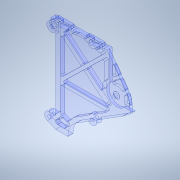
# Autodesk Inventor part: 後ろウィング固定フレームver2(ミラー)
Saved by Autodesk Inventor 2020.2 (Build 242310000, 310)
## iProperties
Created: 2020-05-07
Part Number: 後ろウィング固定フレームver2(ミラー)
Material: ポリカーボネート、クリア
Document SubType Name: Modeling
Designer: mozar
Density: 1.2 g/cm^3
Appearance: ポリカーボネート - クリア
Mass: 16.2166 g
Surface Area: 139.125 cm^2
Volume: 13.5139 cm^3
Author: mozar
Autodesk Inventor part; units mm, degrees
(part 1 of 4)
ref_plane "YZ Plane" through (0, 0, 0) normal (1, 0, 0) x (0, 1, 0)
ref_plane "XZ Plane" through (0, 0, 0) normal (0, 1, 0) x (-1, 0, 0)
ref_plane "XY Plane" through (0, 0, 0) normal (0, 0, 1) x (1, 0, 0)
sketch "スケッチ1" plane through (0, 0, 0) normal (0, 0, 1) x (1, 0, 0)
  line L0 (-101.5, 48) -> (108.5, 48)
  circle A0 centre (111.885, -39) radius 4
  circle A1 centre (191.8767, -37.843) radius 4
  circle A2 centre (111.885, -39) radius 7
  circle A3 centre (191.8767, -37.843) radius 7
  line L1 (191.8767, -37.843) -> (111.885, -39) construction
  line L2 (191.7754, -30.8437) -> (111.7838, -32.0007)
  line L3 (111.9863, -45.9993) -> (191.9779, -44.8422)
  arc A4 (191.9779, -44.8422) -> (191.7754, -30.8437) centre (191.8767, -37.843) ccw
  arc A5 (111.7838, -32.0007) -> (111.9863, -45.9993) centre (111.885, -39) ccw
  line L4 (193.5423, -31.044) -> (241.7048, -42.843)
  circle A6 centre (234.5664, -71.9813) radius 30
  line L5 (262.5874, -82.6971) -> (213.7253, -50.4025)
  line L6 (213.7253, -50.4025) -> (190.2111, -44.6419)
  line L7 (264.5664, -121.5429) -> (264.5664, -63.2267)
  line L8 (111.885, -39) -> (111.885, 41) construction
  line L9 (118.885, -39) -> (118.885, 41)
  line L10 (104.885, 41) -> (104.885, -39)
  arc A7 (104.885, -39) -> (118.885, -39) centre (111.885, -39) ccw
  arc A8 (118.885, 41) -> (104.885, 41) centre (111.885, 41) ccw
  circle A9 centre (58.2383, 51.482) radius 30
  line L11 (113.5581, 34.2029) -> (65.4084, 22.3514)
  line L12 (28.4411, 48) -> (86.7041, 42.0109)
  line L13 (86.7041, 42.0109) -> (110.212, 47.7971)
  circle A10 centre (113.5, -20) radius 68
  line L14 (315.3272, -100.5855) -> (70.6004, 104.7647)
  line L15 (253.8501, -49) -> (111.885, -39)
  arc A11 (93.5924, -27.1048) -> (135.371, -5.9244) centre (95.0604, 21.7941) ccw
  arc A12 (135.371, -5.9244) -> (135.8476, -3.6716) centre (132.899, -4.2246) ccw
  arc A13 (135.8476, -3.6716) -> (83.1833, 18.5565) centre (102.1579, -9.9896) ccw
  line L16 (111.885, -39) -> (112.7472, 40.9954) construction
  line L17 (118.8846, -39.0754) -> (119.7468, 40.9199)
  line L18 (105.7476, 41.0708) -> (104.8855, -38.9246)
  arc A14 (104.8855, -38.9246) -> (118.8846, -39.0754) centre (111.885, -39) ccw
  arc A15 (119.7468, 40.9199) -> (105.7476, 41.0708) centre (112.7472, 40.9954) ccw
  line L19 (164.9949, 48) -> (164.9949, 26)
  line L20 (164.9949, 26) -> (327.4949, -102)
  circle A16 centre (116.2926, -40) radius 68
  circle A17 centre (-98.885, 0) radius 67.5
  line L21 (321.3633, -8.501) -> (-152.6681, 78.4982)
  line L22 (104.8897, -3) -> (104.8897, 0)
  line L23 (104.8897, -3) -> (64.4443, -3)
  line L24 (72.0656, 0) -> (104.8897, 0)
  circle A18 centre (83.3769, -17.5) radius 13.85
  line L25 (198.5102, -35.6076) -> (190.7791, -12.6656)
  line L26 (185.2432, -40.0784) -> (169.4082, 6.912)
  circle A19 centre (197.8374, 16.4922) radius 30
  line L27 (190.7791, -12.6656) -> (191.8767, 45.8941)
  circle A20 centre (191.8767, -37.843) radius 83.7371
  line L28 (191.8767, 45.8941) -> (191.8767, -37.843)
  line L29 (96.8897, -3) -> (96.8897, -6)
  line L30 (96.8897, -6) -> (87.8897, -6)
  line L31 (87.8897, -6) -> (87.8897, -3)
  line L32 (76.4443, -3) -> (76.4443, -6)
  line L33 (76.4443, -6) -> (67.4443, -6)
  line L34 (67.4443, -6) -> (67.4443, -3)
  line L35 (99.8897, -3) -> (99.8897, 0)
  line L36 (99.8897, 0) -> (84.8897, 0)
  line L37 (84.8897, 0) -> (84.8897, -3)
  line L38 (79.4443, -3) -> (79.4443, 0)
  line L39 (79.4443, 0) -> (64.4443, 0)
  line L40 (64.4443, 0) -> (64.4443, -3)
  line L41 (64.4443, 0) -> (59.4443, 0)
  line L42 (59.4443, 0) -> (59.4443, -3)
  line L43 (59.4443, -3) -> (64.4443, -3)
  line L44 (59.4443, -3) -> (59.4443, -6)
  circle A21 centre (111.885, -39) radius 1.5
  circle A22 centre (111.885, -39) radius 9
  circle A23 centre (111.885, -39) radius 10
  circle A24 centre (111.885, -39) radius 15
  line L45 (121.0577, -50.8686) -> (142.9273, -50.5523)
  line L46 (121.0577, -50.8686) -> (127.6513, -45.7727)
  line L47 (127.6513, -45.7727) -> (126.8081, -37.4821)
  line L48 (124.1514, -30.3665) -> (104.8897, -3)
  line L49 (101.0602, -49.3838) -> (59.4443, -6)
  circle A25 centre (95.8897, -6) radius 1
  circle A26 centre (88.8897, -6) radius 1
  circle A27 centre (95.8897, -3) radius 1
  circle A28 centre (88.8897, -3) radius 1
  circle A29 centre (100.8897, -3) radius 1
  circle A30 centre (83.8897, -3) radius 1
  circle A31 centre (80.4443, -3) radius 1
  circle A32 centre (75.4443, -6) radius 1
  circle A33 centre (68.4443, -6) radius 1
  circle A34 centre (75.4443, -3) radius 1
  circle A35 centre (68.4443, -3) radius 1
  circle A36 centre (63.4443, -3) radius 1
  point P0 (0, 0)
  point P1 (151.8809, -38.4215)
  point P2 (111.885, 1)
  point P3 (105.885, 0)
  point P4 (105.885, 0)
  point P5 (23.7328, -42.729)
  point P6 (112.3161, 0.9977)
  point P7 (99.8897, -1.5)
  point P8 (76.4443, -4.5)
  point P9 (74.4443, -6)
  point P10 (69.4443, -6)
  point P11 (69.4443, -3)
  point P12 (74.4443, -3)
  point P13 (82.8897, -3)
  point P14 (81.4443, -3)
  point P15 (62.4443, -3)
  point P16 (101.8897, -3)
  point P17 (89.8897, -3)
  point P18 (94.8897, -3)
  point P19 (94.8897, -6)
  point P20 (89.8897, -6)
  point P21 (118.9616, -31.9344)
  point P22 (118.9245, -31.8974)
  point P23 (118.962, -31.8969)
  point P24 (119.127, -45.896)
  point P25 (104.885, -3)
  point P26 (104.885, -31.8586)
  dimension "d27" = 167.4741
  dimension "d0" = 8
  dimension "d1" = 8
  dimension "d2" = 3
  dimension "d3" = 3
  dimension "d4" = 80
  dimension "d5" = 14
  dimension "d6" = 14
  dimension "d7" = 60
  dimension "d8" = 14
  dimension "d9" = 60
  dimension "d10" = 14
  dimension "d11" = 6
  dimension "d12" = 40
  dimension "d13" = 13.271
  dimension "d14" = 14
  dimension "d15" = 10
  dimension "d16" = 5
  dimension "d17" = 22
  dimension "d18" = 150
  dimension "d19" = 162.5
  dimension "d20" = 0
  dimension "d21" = 136
  dimension "d22" = 136
  dimension "d23" = 135
  dimension "d24" = 38.227
  dimension "d25" = 25
  dimension "d26" = 60
  dimension "d28" = 5
  dimension "d29" = 3
  dimension "d30" = 5
  dimension "d31" = 3
  dimension "d32" = 3
  dimension "d33" = 5
  dimension "d34" = 1
  dimension "d35" = 5
  dimension "d36" = 5
  dimension "d37" = 2
  dimension "d38" = 2
  dimension "d39" = 2
  dimension "d40" = 2
  dimension "d41" = 2
  dimension "d42" = 2
  dimension "d43" = 2
  dimension "d44" = 2
  dimension "d45" = 2
  dimension "d46" = 2
  dimension "d47" = 2
  dimension "d48" = 2
  constraints: 104 end point, 46 tangent, 37 point on circle, 36 centre point, 14 vertical, 8 point on line, 7 equal length, 7 horizontal, 5 coincident, 5 midpoint, 5 parallel, 1 concentric, 1 perpendicular, 1 vertical alignment, 25 other
  measures "d0" diameter of A0
  measures "d1" diameter of A1
  measures "d2" radial gap between concentric circles of A0 A2
  measures "d3" radial gap between concentric circles of A1 A3
  measures "d4" distance of L1.start L1.end
  measures "d5" diameter of A5
  measures "d6" distance from line of L4 L5.end
  measures "d7" diameter of A6
  measures "d8" diameter of A8
  measures "d9" diameter of A9
  measures "d10" distance from line of L11 L12.end
  measures "d11" horizontal distance of L1.end point (105.885, 0)
  measures "d12" angle of L14 L0
  measures "d14" diameter of A15
  measures "d15" vertical distance of L15.start L1.end
  measures "d16" vertical distance of L1.start L4.end
  measures "d17" distance of L19.start L19.end
  measures "d18" vertical distance of L19.start L20.end
  measures "d19" distance from line of L19 L20.end
  measures "d20" distance from line of L19.start L0
  measures "d21" diameter of A10
  measures "d22" diameter of A16
  measures "d23" diameter of A17
  measures "d24" angle of L0 L20
  measures "d25" distance from line of L5.start L20
  measures "d26" diameter of A19
  measures "d28" distance between parallel lines of L35 L22
  measures "d29" distance of L41.end L42.end
  measures "d30" distance of L42.end L40.end
  measures "d31" distance of L42.end L44.end
  measures "d32" diameter of A21
  measures "d33" radial gap between concentric circles of A0 A22
  measures "d34" radial gap between concentric circles of A22 A23
  measures "d35" radial gap between concentric circles of A23 A24
  measures "d36" distance between parallel lines of L3 L45
  measures "d37" diameter of A25
  measures "d38" diameter of A26
  measures "d39" diameter of A27
  measures "d40" diameter of A28
  measures "d41" diameter of A29
  measures "d42" diameter of A30
  measures "d43" diameter of A31
  measures "d44" diameter of A32
  measures "d45" diameter of A33
  measures "d46" diameter of A34
  measures "d47" diameter of A35
  measures "d48" diameter of A36
extrude "押し出し1" add sketch "スケッチ1" against normal blind 5 contours A24 A11 L10 A23 A20 | A20 A23 L3 A24 | L43 A36 L23 L34 A33 L33 A32 A18 L49 L44 | L46 A24 L3 | L3 A24 L15 L47 | A23 L10 A22 A20 | A20 A22 L3 A23 | L49 A18 L30 A25 L29 L23 A29 L10 A24 | L39 L24 L38 L23 A34 A35 L40 | L3 A23 L15 A24 | L15 A24 L47 | A22 L10 A2 A20 | A20 A2 L3 A22 | A23 L18 A22 L10 | L10 A11 L18 A23 | L3 A22 L15 A23 | A24 L10 A11 | L49 A18 A32 L32 A31 A30 L31 A26 L30 | L15 A23 L17 L2 A24 | L2 L17 A24 | A20 A0 L15 A2 | A2 A20 A0 | A22 L18 L10 | L3 A2 L15 A22 | L10 A24 L18 A11 | A23 A20 A22 L18 | L18 A11 A20 A23 | L15 A22 L17 A23 | L10 L23 L48 L18 A24 | L35 L23 A27 A28 L37 L24 | L48 A20 A24 L18 | L17 A23 L2 | L2 A23 L9 A24 L17 | A24 L17 L48 | A20 A0 | A0 A20 | L18 A22 A20 A2 | L15 A2 L17 A22 | L18 A24 A20 A11 | A23 L9 L2 A22 A20 | A20 A11 A24 L9 A23 | A31 A18 L32 L23 | L48 A11 A24 A20 | A23 L17 A22 L9 L2 | L2 L9 A23 | A24 L9 L48 L17 | L15 A0 A20 A2 | A20 A22 L2 A2 | A20 A24 A11 | A18 A30 L23 L31 | L23 A30 A18 A31 | L48 L9 A24 A11 | L9 A22 L2 | L17 L9 A22 | L2 A22 L9 A2
extrude "押し出し2" cut sketch "スケッチ1" against normal blind 2.55 contours L3 A24 L15 L47 | A23 L10 A22 A20 | A20 A22 L3 A23 | L3 A23 L15 A24 | L15 A24 L47 | A22 L10 A2 A20 | A20 A2 L3 A22 | A23 L18 A22 L10 | L10 A11 L18 A23 | L3 A22 L15 A23 | L15 A23 L17 L2 A24 | L2 L17 A24 | A20 A0 L15 A2 | A2 A20 A0 | A22 L18 L10 | L3 A2 L15 A22 | L10 A24 L18 A11 | A23 A20 A22 L18 | L18 A11 A20 A23 | L15 A22 L17 A23 | L10 L23 L48 L18 A24 | L48 A20 A24 L18 | L17 A23 L2 | L2 A23 L9 A24 L17 | A24 L17 L48 | A20 A0 | A0 A20 | L18 A22 A20 A2 | L15 A2 L17 A22 | L18 A24 A20 A11 | A23 L9 L2 A22 A20 | A20 A11 A24 L9 A23 | L48 A11 A24 A20 | A23 L17 A22 L9 L2 | L2 L9 A23 | A24 L9 L48 L17 | L15 A0 A20 A2 | A20 A22 L2 A2 | A20 A24 A11 | L48 L9 A24 A11 | L9 A22 L2 | L17 L9 A22 | L2 A22 L9 A2 | A21
sketch "スケッチ2" plane through (0, 0, 0) normal (0, 0, 1) x (1, 0, 0)
  line L0 (87.8897, -6) -> (87.8897, -3) projected
  arc A0 (89.8897, -3) -> (87.8897, -3) centre (88.8897, -3) ccw projected
  line L1 (89.8897, -3) -> (94.8897, -3) projected
  arc A1 (96.8897, -3) -> (94.8897, -3) centre (95.8897, -3) ccw projected
  line L2 (96.8897, -3) -> (96.8897, -6) projected
  arc A2 (94.8897, -6) -> (96.8897, -6) centre (95.8897, -6) ccw projected
  line L3 (94.8897, -6) -> (89.8897, -6) projected
  arc A3 (87.8897, -6) -> (89.8897, -6) centre (88.8897, -6) ccw projected
  arc A4 (67.4443, -6) -> (69.4443, -6) centre (68.4443, -6) ccw projected
  line L4 (67.4443, -6) -> (67.4443, -3) projected
  arc A5 (69.4443, -3) -> (67.4443, -3) centre (68.4443, -3) ccw projected
  line L5 (69.4443, -3) -> (74.4443, -3) projected
  arc A6 (76.4443, -3) -> (74.4443, -3) centre (75.4443, -3) ccw projected
  line L6 (76.4443, -3) -> (76.4443, -6) projected
  arc A7 (74.4443, -6) -> (76.4443, -6) centre (75.4443, -6) ccw projected
  line L7 (74.4443, -6) -> (69.4443, -6) projected
  line L8 (127.6513, -45.7727) -> (119.127, -45.896) projected
  arc A8 (104.885, -31.8586) -> (119.127, -45.896) centre (111.885, -39) ccw projected
  line L9 (104.885, -31.8586) -> (104.885, -3) projected
  line L10 (104.885, -3) -> (101.8897, -3) projected
  arc A9 (99.8897, -3) -> (101.8897, -3) centre (100.8897, -3) ccw projected
  line L11 (99.8897, -3) -> (99.8897, 0) projected
  line L12 (99.8897, 0) -> (84.8897, 0) projected
  line L13 (84.8897, 0) -> (84.8897, -3) projected
  arc A10 (82.8897, -3) -> (84.8897, -3) centre (83.8897, -3) ccw projected
  line L14 (82.8897, -3) -> (81.4443, -3) projected
  arc A11 (79.4443, -3) -> (81.4443, -3) centre (80.4443, -3) ccw projected
  line L15 (79.4443, -3) -> (79.4443, 0) projected
  line L16 (79.4443, 0) -> (64.4443, 0) projected
  line L17 (64.4443, 0) -> (64.4443, -3) projected
  arc A12 (62.4443, -3) -> (64.4443, -3) centre (63.4443, -3) ccw projected
  line L18 (62.4443, -3) -> (59.4443, -3) projected
  line L19 (59.4443, -3) -> (59.4443, -6) projected
  line L20 (59.4443, -6) -> (101.0602, -49.3838) projected
  arc A13 (101.0602, -49.3838) -> (121.0577, -50.8686) centre (111.885, -39) ccw projected
  line L21 (121.0577, -50.8686) -> (127.6513, -45.7727) projected
  circle A14 centre (111.885, -39) radius 1.5 projected
  circle A15 centre (111.885, -39) radius 3
  point P0 (0, 0)
  dimension "d53" = 6
  constraints: 1 centre point, 1 coincident
  measures "d53" diameter of A15
extrude "押し出し3" cut sketch "スケッチ2" against normal blind 3 contours A15
sketch "スケッチ3" plane through (0, 0, 0) normal (0, 0, 1) x (1, 0, 0)
  line L0 (87.8897, -6) -> (87.8897, -3) projected
  arc A0 (89.8897, -3) -> (87.8897, -3) centre (88.8897, -3) ccw projected
  line L1 (89.8897, -3) -> (94.8897, -3) projected
  arc A1 (96.8897, -3) -> (94.8897, -3) centre (95.8897, -3) ccw projected
  line L2 (96.8897, -3) -> (96.8897, -6) projected
  arc A2 (94.8897, -6) -> (96.8897, -6) centre (95.8897, -6) ccw projected
  line L3 (94.8897, -6) -> (89.8897, -6) projected
  arc A3 (87.8897, -6) -> (89.8897, -6) centre (88.8897, -6) ccw projected
  arc A4 (67.4443, -6) -> (69.4443, -6) centre (68.4443, -6) ccw projected
  line L4 (67.4443, -6) -> (67.4443, -3) projected
  arc A5 (69.4443, -3) -> (67.4443, -3) centre (68.4443, -3) ccw projected
  line L5 (69.4443, -3) -> (74.4443, -3) projected
  arc A6 (76.4443, -3) -> (74.4443, -3) centre (75.4443, -3) ccw projected
  line L6 (76.4443, -3) -> (76.4443, -6) projected
  arc A7 (74.4443, -6) -> (76.4443, -6) centre (75.4443, -6) ccw projected
  line L7 (74.4443, -6) -> (69.4443, -6) projected
  line L8 (127.6513, -45.7727) -> (119.127, -45.896) projected
  arc A8 (104.885, -31.8586) -> (119.127, -45.896) centre (111.885, -39) ccw projected
  line L9 (104.885, -31.8586) -> (104.885, -3) projected
  line L10 (104.885, -3) -> (101.8897, -3) projected
  arc A9 (99.8897, -3) -> (101.8897, -3) centre (100.8897, -3) ccw projected
  line L11 (99.8897, -3) -> (99.8897, 0) projected
  line L12 (99.8897, 0) -> (84.8897, 0) projected
  line L13 (84.8897, 0) -> (84.8897, -3) projected
  arc A10 (82.8897, -3) -> (84.8897, -3) centre (83.8897, -3) ccw projected
  line L14 (82.8897, -3) -> (81.4443, -3) projected
  arc A11 (79.4443, -3) -> (81.4443, -3) centre (80.4443, -3) ccw projected
  line L15 (79.4443, -3) -> (79.4443, 0) projected
  line L16 (79.4443, 0) -> (64.4443, 0) projected
  line L17 (64.4443, 0) -> (64.4443, -3) projected
  arc A12 (62.4443, -3) -> (64.4443, -3) centre (63.4443, -3) ccw projected
  line L18 (62.4443, -3) -> (59.4443, -3) projected
  line L19 (59.4443, -3) -> (59.4443, -6) projected
  line L20 (59.4443, -6) -> (101.0602, -49.3838) projected
  arc A13 (101.0602, -49.3838) -> (121.0577, -50.8686) centre (111.885, -39) ccw projected
  line L21 (121.0577, -50.8686) -> (127.6513, -45.7727) projected
  line L22 (99.8897, 0) -> (99.8897, -3) projected
  line L23 (99.8897, 0) -> (64.4443, 0)
  line L24 (64.4443, 0) -> (64.4443, -3)
  line L25 (64.4443, -3) -> (99.8897, -3)
  line L26 (99.8897, -3) -> (99.8897, 0)
  point P0 (0, 0)
  constraints: 8 end point, 2 parallel, 1 horizontal, 1 perpendicular
extrude "押し出し4" cut sketch "スケッチ3" against normal blind 2 contours L25 L13 L12 L11 A1 L1 A0 | A0 L25 | L25 L14 L15 L23 L13 | A1 L25 | L15 L25 A6 L5 A5 L17 L16 | L25 A6 | A5 L25
sketch "スケッチ4" plane through (0, 0, -5) normal (0, 0, -1) x (-1, 0, 0)
  circle A0 centre (-111.885, -39) radius 3 projected
  line L0 (-104.885, -3) -> (-104.8897, -3) projected
  line L1 (-104.885, -31.8586) -> (-104.885, -3) projected
  arc A1 (-119.127, -45.896) -> (-104.885, -31.8586) centre (-111.885, -39) ccw projected
  line L2 (-127.6513, -45.7727) -> (-119.127, -45.896) projected
  line L3 (-126.8081, -37.4821) -> (-127.6513, -45.7727) projected
  arc A2 (-124.1514, -30.3665) -> (-126.8081, -37.4821) centre (-111.885, -39) ccw projected
  line L4 (-104.8897, -3) -> (-124.1514, -30.3665) projected
  circle A3 centre (-111.885, -39) radius 1.5 projected
  point P0 (0, 0)
sketch "スケッチ5" plane through (0, 0, 0) normal (0, 0, 1) x (1, 0, 0)
  circle A0 centre (111.885, -39) radius 3 projected
  line L0 (104.885, -3) -> (104.8897, -3) projected
  line L1 (104.885, -31.8586) -> (104.885, -3) projected
  arc A1 (104.885, -31.8586) -> (119.127, -45.896) centre (111.885, -39) ccw projected
  line L2 (127.6513, -45.7727) -> (119.127, -45.896) projected
  line L3 (126.8081, -37.4821) -> (127.6513, -45.7727) projected
  arc A2 (126.8081, -37.4821) -> (124.1514, -30.3665) centre (111.885, -39) ccw projected
  line L4 (104.8897, -3) -> (124.1514, -30.3665) projected
  circle A3 centre (111.885, -39) radius 1.5 projected
  point P0 (0, 0)
extrude "押し出し5" add sketch "スケッチ5" against normal blind 3 contours A0 | L0 L4 A2 L3 L2 A1 L1
extrude "押し出し6" cut sketch "スケッチ4" against normal blind 3 contours A0
extrude "押し出し7" cut sketch "スケッチ4" against normal blind 2.55 contours L1 A1 L2 L3 A2 L4 L0
sketch "スケッチ6" plane through (0, 0, -5) normal (0, 0, -1) x (-1, 0, 0)
  line L0 (-79.4443, 0) -> (-79.4443, -3) projected
  line L1 (-64.4443, 0) -> (-79.4443, 0) projected
  line L2 (-64.4443, -3) -> (-64.4443, 0) projected
  line L3 (-67.4443, -3) -> (-64.4443, -3) projected
  arc A0 (-67.4443, -3) -> (-69.4443, -3) centre (-68.4443, -3) ccw projected
  line L4 (-74.4443, -3) -> (-69.4443, -3) projected
  arc A1 (-74.4443, -3) -> (-76.4443, -3) centre (-75.4443, -3) ccw projected
  line L5 (-79.4443, -3) -> (-76.4443, -3) projected
  arc A2 (-94.8897, -3) -> (-96.8897, -3) centre (-95.8897, -3) ccw projected
  line L6 (-99.8897, -3) -> (-96.8897, -3) projected
  line L7 (-99.8897, 0) -> (-99.8897, -3) projected
  line L8 (-84.8897, 0) -> (-99.8897, 0) projected
  line L9 (-84.8897, -3) -> (-84.8897, 0) projected
  line L10 (-87.8897, -3) -> (-84.8897, -3) projected
  arc A3 (-87.8897, -3) -> (-89.8897, -3) centre (-88.8897, -3) ccw projected
  line L11 (-94.8897, -3) -> (-89.8897, -3) projected
  point P0 (0, 0)
sketch "スケッチ7" plane through (0, 0, 0) normal (0, 0, 1) x (1, 0, 0)
  arc A0 (96.8897, -3) -> (94.8897, -3) centre (95.8897, -3) ccw projected
  line L0 (99.8897, -3) -> (96.8897, -3) projected
  line L1 (99.8897, 0) -> (99.8897, -3) projected
  line L2 (84.8897, 0) -> (99.8897, 0) projected
  line L3 (84.8897, -3) -> (84.8897, 0) projected
  line L4 (87.8897, -3) -> (84.8897, -3) projected
  arc A1 (89.8897, -3) -> (87.8897, -3) centre (88.8897, -3) ccw projected
  line L5 (94.8897, -3) -> (89.8897, -3) projected
  line L6 (79.4443, 0) -> (79.4443, -3) projected
  line L7 (64.4443, 0) -> (79.4443, 0) projected
  line L8 (64.4443, -3) -> (64.4443, 0) projected
  line L9 (67.4443, -3) -> (64.4443, -3) projected
  arc A2 (69.4443, -3) -> (67.4443, -3) centre (68.4443, -3) ccw projected
  line L10 (74.4443, -3) -> (69.4443, -3) projected
  arc A3 (76.4443, -3) -> (74.4443, -3) centre (75.4443, -3) ccw projected
  line L11 (79.4443, -3) -> (76.4443, -3) projected
  point P0 (0, 0)
extrude "押し出し8" add sketch "スケッチ7" against normal blind 5
extrude "押し出し9" cut sketch "スケッチ6" against normal blind 2
sketch "スケッチ8" plane through (0, 0, -5) normal (0, 0, -1) x (-1, 0, 0)
  line L0 (-84.8897, -3) -> (-87.8897, -3) projected
  line L1 (-87.8897, -3) -> (-87.8897, -6) projected
  arc A0 (-89.8897, -6) -> (-87.8897, -6) centre (-88.8897, -6) ccw projected
  line L2 (-89.8897, -6) -> (-94.8897, -6) projected
  arc A1 (-96.8897, -6) -> (-94.8897, -6) centre (-95.8897, -6) ccw projected
  line L3 (-96.8897, -6) -> (-96.8897, -3) projected
  line L4 (-96.8897, -3) -> (-99.8897, -3) projected
  arc A2 (-101.8897, -3) -> (-99.8897, -3) centre (-100.8897, -3) ccw projected
  line L5 (-101.8897, -3) -> (-104.885, -3) projected
  line L6 (-104.885, -3) -> (-104.885, -31.8586) projected
  arc A3 (-119.127, -45.896) -> (-104.885, -31.8586) centre (-111.885, -39) ccw projected
  line L7 (-119.127, -45.896) -> (-127.6513, -45.7727) projected
  line L8 (-127.6513, -45.7727) -> (-121.0577, -50.8686) projected
  arc A4 (-121.0577, -50.8686) -> (-101.0602, -49.3838) centre (-111.885, -39) ccw projected
  line L9 (-101.0602, -49.3838) -> (-59.4443, -6) projected
  line L10 (-59.4443, -6) -> (-59.4443, -3) projected
  line L11 (-59.4443, -3) -> (-62.4443, -3) projected
  arc A5 (-64.4443, -3) -> (-62.4443, -3) centre (-63.4443, -3) ccw projected
  line L12 (-64.4443, -3) -> (-67.4443, -3) projected
  line L13 (-67.4443, -3) -> (-67.4443, -6) projected
  arc A6 (-69.4443, -6) -> (-67.4443, -6) centre (-68.4443, -6) ccw projected
  line L14 (-69.4443, -6) -> (-74.4443, -6) projected
  arc A7 (-76.4443, -6) -> (-74.4443, -6) centre (-75.4443, -6) ccw projected
  line L15 (-76.4443, -6) -> (-76.4443, -3) projected
  line L16 (-76.4443, -3) -> (-79.4443, -3) projected
  arc A8 (-81.4443, -3) -> (-79.4443, -3) centre (-80.4443, -3) ccw projected
  line L17 (-81.4443, -3) -> (-82.8897, -3) projected
  arc A9 (-84.8897, -3) -> (-82.8897, -3) centre (-83.8897, -3) ccw projected
  line L18 (-66.4443, -6) -> (-57.4443, -6)
  line L19 (-57.4443, -6) -> (-57.4443, -3)
  line L20 (-57.4443, -3) -> (-66.4443, -3)
  line L21 (-66.4443, -3) -> (-66.4443, -6)
  line L22 (-69.4443, -6) -> (-74.4443, -6) projected
  line L23 (-64.4443, -3) -> (-67.4443, -3) projected
  circle A10 centre (-65.4443, -3) radius 1
  circle A11 centre (-65.4443, -6) radius 1
  circle A12 centre (-58.4443, -3) radius 1
  circle A13 centre (-58.4443, -6) radius 1
  line L24 (-54.4443, 0) -> (-54.4443, -6)
  line L25 (-61.0901, -9) -> (-62.7986, -9)
  line L26 (-69.4443, -6) -> (-69.4443, 0)
  line L27 (-69.4443, 0) -> (-54.4443, 0)
  circle A14 centre (-65.4443, -6) radius 4
  circle A15 centre (-58.4443, -6) radius 4
  line L28 (-64.4443, 0) -> (-64.4443, -3) projected
  line L29 (-79.4443, -3) -> (-79.4443, 0) projected
  line L30 (-69.4443, 0) -> (-54.4443, 0)
  line L31 (-54.4443, 0) -> (-54.4443, -3)
  line L32 (-54.4443, -3) -> (-69.4443, -3)
  line L33 (-69.4443, -3) -> (-69.4443, 0)
  line L34 (-54.4443, -3) -> (-49.4443, -3)
  line L35 (-49.4443, -3) -> (-49.4443, -6)
  line L36 (-49.4443, -6) -> (-54.4443, -6)
  line L37 (-54.4443, -6) -> (-54.4443, -3)
  circle A16 centre (-53.4443, -3) radius 1
  circle A17 centre (-70.4443, -3) radius 1
  line L38 (-76.4443, -3) -> (-69.4443, -3)
  line L39 (-79.4443, 0) -> (-64.4443, 0) projected
  line L40 (-79.4443, 0) -> (-64.4443, 0)
  line L41 (-81.4443, -3) -> (-79.4443, -3)
  point P0 (0, 0)
  point P1 (-61.9443, -3)
  point P2 (-52.4443, -3)
  point P3 (-71.4443, -3)
  point P4 (-59.4443, -6)
  point P5 (-64.4443, -6)
  dimension "d68" = 9
  dimension "d69" = 3
  dimension "d70" = 10
  dimension "d71" = 2
  dimension "d72" = 2
  dimension "d73" = 2
  dimension "d74" = 2
  dimension "d75" = 3
  dimension "d76" = 3
  dimension "d77" = 3
  dimension "d78" = 3
  dimension "d79" = 15
  dimension "d80" = 15
  dimension "d81" = 3
  dimension "d82" = 3
  dimension "d83" = 15
  dimension "d84" = 3
  dimension "d85" = 10
  dimension "d86" = 2
  dimension "d88" = 2
  constraints: 38 end point, 8 centre point, 8 parallel, 7 point on line, 7 tangent, 4 horizontal, 4 perpendicular, 4 point on circle, 2 midpoint, 1 collinear
  measures "d68" distance of L20.end L19.end
  measures "d69" distance of L19.end L18.end
  measures "d70" distance between parallel lines of L15 L21
  measures "d71" diameter of A10
  measures "d72" diameter of A11
  measures "d73" diameter of A12
  measures "d74" diameter of A13
  measures "d75" distance between parallel lines of L19 L24
  measures "d76" radial gap between concentric circles of A11 A14
  measures "d77" radial gap between concentric circles of A13 A15
  measures "d78" distance between parallel lines of L14 L25
  measures "d79" distance between parallel lines of L28 L29
  measures "d80" distance of L31.end L32.end
  measures "d81" distance of L30.end L31.end
  measures "d82" distance between parallel lines of L32 L27
  measures "d83" distance between parallel lines of L31 L33
  measures "d84" distance of L34.end L35.end
  measures "d85" distance between parallel lines of L35 L10
  measures "d86" diameter of A16
  measures "d88" diameter of A17
extrude "押し出し10" cut sketch "スケッチ8" against normal blind 10 contours L29 L39 L26 A17 L38 L16 | A17 L38 | L27 L28 A14 L32 L26 | A14 A10 L12 L32 | L28 A10 A14 | A10 L12 picked at (-70.1948, -2.6194) picked at (-65.2365, -2.4501)
extrude "押し出し11" add sketch "スケッチ8" against normal blind 5 contours L38 A17 L26 L14 A7 L15 | L27 L28 A14 L32 L26 | L32 A14 L26 | L27 L24 L32 A15 L11 L20 A14 L28 | A14 L32 L13 A6 | A6 L13 L12 L21 A11 L18 A15 A14 | A14 A10 L12 L32 | L28 A10 A14 | A14 L20 L28 | A14 A15 L9 L25 | A10 L12 | A16 L34 L35 L36 L24 | L24 A15 L32 | A14 A5 L20 | L20 A5 A14 | A10 L12 | A5 A14 A15 L18 A11 L21 A10 | L9 A15 L25 | A15 L18 A14 | A14 L18 L9 A15 | A15 L9 A13 L19 L32 | L32 A12 A15 | L11 A15 A14 A5 | A14 A15 L11 L10 L18 | L18 A15 A14 | A12 L20 | A12 L11 A15 | A12 L20 | L19 A13 L10 A12 | A13 L18 | L18 A13
extrude "押し出し12" cut sketch "スケッチ8" against normal blind 10 contours A10 L12 | A14 A5 L20 | L20 A5 A14 | A10 L12 | A5 A14 A15 L18 A11 L21 A10 | L11 A15 A14 A5 | A14 A15 L11 L10 L18 | L18 A15 A14 | A11 L18 | L18 A11 | A12 L20 | A12 L20 | L19 A13 L10 A12 | A13 L18 | L18 A13 picked at (-61.7965, -5.7765)
extrude "押し出し13" add sketch "スケッチ8" against normal blind 5 contours L41 A8
sketch "スケッチ9" plane through (0, 0, -5) normal (0, 0, -1) x (-1, 0, 0)
  line L0 (-59.4443, -6) -> (-64.4443, -6) projected
  arc A0 (-66.4443, -6) -> (-64.4443, -6) centre (-65.4443, -6) ccw projected
  line L1 (-66.4443, -6) -> (-66.4443, -3) projected
  arc A1 (-64.4443, -3) -> (-66.4443, -3) centre (-65.4443, -3) ccw projected
  line L2 (-64.4443, -3) -> (-59.4443, -3) projected
  arc A2 (-57.4443, -3) -> (-59.4443, -3) centre (-58.4443, -3) ccw projected
  line L3 (-57.4443, -3) -> (-57.4443, -6) projected
  arc A3 (-59.4443, -6) -> (-57.4443, -6) centre (-58.4443, -6) ccw projected
  line L4 (-62.3221, -9) -> (-61.0901, -9) projected
  arc A4 (-61.0901, -9) -> (-54.4443, -6) centre (-58.4443, -6) ccw projected
  line L5 (-54.4443, -6) -> (-49.4443, -6) projected
  line L6 (-49.4443, -6) -> (-49.4443, -3) projected
  line L7 (-49.4443, -3) -> (-52.4443, -3) projected
  arc A5 (-54.4443, -3) -> (-52.4443, -3) centre (-53.4443, -3) ccw projected
  line L8 (-54.4443, -3) -> (-54.4443, 0) projected
  line L9 (-54.4443, 0) -> (-69.4443, 0) projected
  line L10 (-69.4443, 0) -> (-69.4443, -3) projected
  arc A6 (-71.4443, -3) -> (-69.4443, -3) centre (-70.4443, -3) ccw projected
  line L11 (-71.4443, -3) -> (-82.8897, -3) projected
  arc A7 (-84.8897, -3) -> (-82.8897, -3) centre (-83.8897, -3) ccw projected
  line L12 (-84.8897, -3) -> (-87.8897, -3) projected
  line L13 (-87.8897, -3) -> (-87.8897, -6) projected
  arc A8 (-89.8897, -6) -> (-87.8897, -6) centre (-88.8897, -6) ccw projected
  line L14 (-89.8897, -6) -> (-94.8897, -6) projected
  arc A9 (-96.8897, -6) -> (-94.8897, -6) centre (-95.8897, -6) ccw projected
  line L15 (-96.8897, -6) -> (-96.8897, -3) projected
  line L16 (-96.8897, -3) -> (-99.8897, -3) projected
  arc A10 (-101.8897, -3) -> (-99.8897, -3) centre (-100.8897, -3) ccw projected
  line L17 (-101.8897, -3) -> (-104.885, -3) projected
  line L18 (-104.885, -3) -> (-104.885, -31.8586) projected
  arc A11 (-119.127, -45.896) -> (-104.885, -31.8586) centre (-111.885, -39) ccw projected
  line L19 (-119.127, -45.896) -> (-127.6513, -45.7727) projected
  line L20 (-127.6513, -45.7727) -> (-121.0577, -50.8686) projected
  arc A12 (-121.0577, -50.8686) -> (-101.0602, -49.3838) centre (-111.885, -39) ccw projected
  line L21 (-101.0602, -49.3838) -> (-62.3221, -9) projected
  circle A13 centre (-111.885, -39) radius 1.5 projected
  line L22 (-101.0602, -49.3838) -> (-62.3221, -9) projected
  circle A14 centre (-111.885, -39) radius 15
  line L23 (-54.4443, -6) -> (-49.4443, -6) projected
  arc A15 (-121.0577, -50.8686) -> (-101.0602, -49.3838) centre (-111.885, -39) ccw projected
  line L24 (-102.2194, -50.4706) -> (-49.4443, -6)
  point P0 (0, 0)
  constraints: 2 end point, 1 coincident, 1 point on circle, 4 other
extrude "押し出し14" add sketch "スケッチ9" against normal blind 5 contours L4 A4 L5 L24 A12 L21
extrude "押し出し15" cut sketch "スケッチ8" against normal blind 2 contours L27 L28 A14 L32 L26 | L27 L24 L32 A15 L11 L20 A14 L28 | A14 A10 L12 L32 | L28 A10 A14 | A14 L20 L28 | A10 L12 | L32 A12 A15 | A12 L20 | A12 L11 A15 picked at (-65.2365, -2.4501) picked at (-58.4443, -2.6667)
sketch "スケッチ10" plane through (0, 0, 0) normal (0, 0, 1) x (1, 0, 0)
  circle A0 centre (111.885, -39) radius 1.5
  circle A1 centre (61.313, -56.1319) radius 13.85
  circle A2 centre (49.8261, -69.3342) radius 1.5
  circle A3 centre (49.8261, -69.3342) radius 3
  circle A4 centre (44.5337, -75.9856) radius 4
  circle A5 centre (61.313, -56.1319) radius 14.5
  circle A6 centre (49.8261, -69.3342) radius 4
  circle A7 centre (44.5337, -75.9856) radius 7
  circle A8 centre (29.9003, -80.4272) radius 2
  circle A9 centre (29.9003, -80.4272) radius 8
  circle A10 centre (31.8401, -37) radius 7.5
  circle A11 centre (31.8401, -37) radius 34
  point P0 (0, 0)
  dimension "d101" = 6
  dimension "d102" = 8
  dimension "d103" = 29
  dimension "d104" = 1
  dimension "d105" = 3
  dimension "d106" = 16
  dimension "d107" = 68
  constraints: 12 centre point, 4 coincident, 2 tangent, 4 other
  measures "d101" diameter of A3
  measures "d102" diameter of A4
  measures "d103" diameter of A5
  measures "d104" radial gap between concentric circles of A3 A6
  measures "d105" radial gap between concentric circles of A4 A7
  measures "d106" diameter of A9
  measures "d107" diameter of A11
sketch "スケッチ11" plane through (0, 0, 0) normal (0, 0, 1) x (1, 0, 0)
  circle A0 centre (111.885, -39) radius 1.5
  circle A1 centre (61.313, -56.1319) radius 13.85
  circle A2 centre (49.8261, -69.3342) radius 1.5
  circle A3 centre (49.8261, -69.3342) radius 3
  circle A4 centre (55.3014, -75.1671) radius 4
  circle A5 centre (61.313, -56.1319) radius 14.5
  circle A6 centre (49.8261, -69.3342) radius 4
  circle A7 centre (55.3014, -75.1671) radius 7
  circle A8 centre (29.9003, -80.4272) radius 2
  circle A9 centre (29.9003, -80.4272) radius 8
  circle A10 centre (31.8401, -37) radius 7.5
  circle A11 centre (31.8401, -37) radius 34
  line L0 (47.463, -56.05) -> (47.463, -31.35)
  line L1 (49.4443, -3) -> (49.4443, -6)
  line L2 (49.4443, -6) -> (49.4443, -63.8313)
  line L3 (54.4443, -63.8313) -> (54.4443, -6)
  line L4 (54.4443, -6) -> (54.4443, -3)
  line L5 (51.3014, -31.35) -> (51.3014, -56.05)
  line L6 (51.3014, -56.05) -> (51.3014, -80.75)
  line L7 (51.3014, -80.75) -> (-20.8943, -80.75)
  point P0 (0, 0)
  dimension "d108" = 6
  dimension "d109" = 8
  dimension "d110" = 29
  dimension "d111" = 1
  dimension "d112" = 3
  dimension "d113" = 16
  dimension "d114" = 68
  dimension "d115" = 5
  constraints: 16 end point, 12 centre point, 5 vertical, 4 coincident, 3 collinear, 2 horizontal, 2 tangent, 5 other
  measures "d108" diameter of A3
  measures "d109" diameter of A4
  measures "d110" diameter of A5
  measures "d111" radial gap between concentric circles of A3 A6
  measures "d112" radial gap between concentric circles of A4 A7
  measures "d113" diameter of A9
  measures "d114" diameter of A11
  measures "d115" distance between parallel lines of L2 L3
sketch "スケッチ12" plane through (0, 0, 0) normal (0, 0, 1) x (1, 0, 0)
  circle A0 centre (111.885, -39) radius 1.5
  circle A1 centre (61.313, -56.1319) radius 13.85
  circle A2 centre (49.8261, -69.3342) radius 1.5
  circle A3 centre (49.8261, -69.3342) radius 3
  circle A4 centre (61.313, -56.1319) radius 14.5
  circle A5 centre (49.8261, -69.3342) radius 4
  circle A6 centre (29.9003, -80.4272) radius 2
  circle A7 centre (29.9003, -80.4272) radius 8
  circle A8 centre (31.8401, -37) radius 7.5
  circle A9 centre (31.8401, -37) radius 34
  line L0 (47.463, -56.05) -> (47.463, -31.35)
  line L1 (49.4443, -3) -> (49.4443, -6)
  line L2 (49.4443, -6) -> (49.4443, -63.8313)
  line L3 (54.3014, -63.8313) -> (54.3014, -6)
  line L4 (54.3014, -6) -> (54.3014, -3)
  line L5 (51.3014, -31.35) -> (51.3014, -56.05)
  line L6 (51.3014, -56.05) -> (51.3014, -80.75)
  line L7 (51.3014, -80.75) -> (-20.8943, -80.75)
  circle A10 centre (61.313, -56.1319) radius 15.85
  line L8 (57.4443, -6) -> (57.4443, -3) projected
  arc A11 (59.4443, -3) -> (57.4443, -3) centre (58.4443, -3) ccw projected
  line L9 (59.4443, -3) -> (64.4443, -3) projected
  arc A12 (66.4443, -3) -> (64.4443, -3) centre (65.4443, -3) ccw projected
  line L10 (66.4443, -3) -> (66.4443, -6) projected
  arc A13 (64.4443, -6) -> (66.4443, -6) centre (65.4443, -6) ccw projected
  line L11 (64.4443, -6) -> (59.4443, -6) projected
  arc A14 (57.4443, -6) -> (59.4443, -6) centre (58.4443, -6) ccw projected
  arc A15 (89.8897, -3) -> (87.8897, -3) centre (88.8897, -3) ccw projected
  line L12 (89.8897, -3) -> (94.8897, -3) projected
  arc A16 (96.8897, -3) -> (94.8897, -3) centre (95.8897, -3) ccw projected
  line L13 (96.8897, -3) -> (96.8897, -6) projected
  arc A17 (94.8897, -6) -> (96.8897, -6) centre (95.8897, -6) ccw projected
  line L14 (94.8897, -6) -> (89.8897, -6) projected
  arc A18 (87.8897, -6) -> (89.8897, -6) centre (88.8897, -6) ccw projected
  line L15 (87.8897, -6) -> (87.8897, -3) projected
  circle A19 centre (111.885, -39) radius 1.5 projected
  arc A20 (102.2194, -50.4706) -> (121.0577, -50.8686) centre (111.885, -39) ccw projected
  line L16 (121.0577, -50.8686) -> (127.6513, -45.7727) projected
  line L17 (127.6513, -45.7727) -> (126.8081, -37.4821) projected
  arc A21 (126.8081, -37.4821) -> (124.1514, -30.3665) centre (111.885, -39) ccw projected
  line L18 (124.1514, -30.3665) -> (104.8897, -3) projected
  line L19 (104.8897, -3) -> (101.8897, -3) projected
  arc A22 (99.8897, -3) -> (101.8897, -3) centre (100.8897, -3) ccw projected
  line L20 (99.8897, -3) -> (99.8897, 0) projected
  line L21 (99.8897, 0) -> (84.8897, 0) projected
  line L22 (84.8897, 0) -> (84.8897, -3) projected
  arc A23 (82.8897, -3) -> (84.8897, -3) centre (83.8897, -3) ccw projected
  line L23 (82.8897, -3) -> (71.4443, -3) projected
  arc A24 (69.4443, -3) -> (71.4443, -3) centre (70.4443, -3) ccw projected
  line L24 (69.4443, -3) -> (69.4443, 0) projected
  line L25 (69.4443, 0) -> (54.4443, 0) projected
  line L26 (54.4443, 0) -> (54.4443, -3) projected
  arc A25 (52.4443, -3) -> (54.4443, -3) centre (53.4443, -3) ccw projected
  line L27 (52.4443, -3) -> (49.4443, -3) projected
  line L28 (49.4443, -3) -> (49.4443, -6) projected
  line L29 (49.4443, -6) -> (102.2194, -50.4706) projected
  line L30 (54.3014, -63.8313) -> (54.3014, -70.0075)
  circle A26 centre (59.4443, -76.68) radius 4
  point P0 (0, 0)
  dimension "d116" = 6
  dimension "d118" = 29
  dimension "d119" = 1
  dimension "d121" = 16
  dimension "d122" = 68
  dimension "d123" = 3
  dimension "d124" = 2
  dimension "d125" = 8
  constraints: 18 end point, 12 centre point, 6 vertical, 4 coincident, 3 collinear, 2 horizontal, 5 other
  measures "d116" diameter of A3
  measures "d118" diameter of A4
  measures "d119" radial gap between concentric circles of A3 A5
  measures "d121" diameter of A7
  measures "d122" diameter of A9
  measures "d123" distance between parallel lines of L3 L5
  measures "d124" radial gap between concentric circles of A1 A10
  measures "d125" diameter of A26
sketch "スケッチ13" plane through (0, 0, 0) normal (0, 0, 1) x (1, 0, 0)
  circle A0 centre (111.885, -39) radius 1.5
  circle A1 centre (61.313, -56.1319) radius 13.85
  circle A2 centre (49.8261, -69.3342) radius 1.5
  circle A3 centre (49.8261, -69.3342) radius 3
  circle A4 centre (44.6461, -90.75) radius 4
  circle A5 centre (61.313, -56.1319) radius 14.5
  circle A6 centre (49.8261, -69.3342) radius 4
  circle A7 centre (44.6461, -90.75) radius 7
  circle A8 centre (29.9003, -80.4272) radius 2
  circle A9 centre (29.9003, -80.4272) radius 8
  circle A10 centre (31.8401, -37) radius 7.5
  circle A11 centre (31.8401, -37) radius 34
  line L0 (47.463, -56.05) -> (47.463, -31.35)
  line L1 (49.4443, -3) -> (49.4443, -6)
  line L2 (49.4443, -6) -> (49.4443, -63.8313)
  line L3 (54.3014, -63.8313) -> (54.3014, -6)
  line L4 (54.3014, -6) -> (54.3014, -3)
  line L5 (51.3014, -31.35) -> (51.3014, -56.05)
  line L6 (51.3014, -56.05) -> (51.3014, -80.75)
  line L7 (51.3014, -80.75) -> (-20.8943, -80.75)
  circle A12 centre (61.313, -56.1319) radius 15.85
  line L8 (-20.8943, -83.75) -> (54.3014, -83.75)
  line L9 (54.3014, -83.75) -> (54.3014, -56.05)
  line L10 (54.3014, -56.05) -> (54.3014, -31.35)
  arc A13 (104.885, -31.8586) -> (119.127, -45.896) centre (111.885, -39) ccw projected
  line L11 (57.4443, -6) -> (57.4443, -3) projected
  arc A14 (59.4443, -3) -> (57.4443, -3) centre (58.4443, -3) ccw projected
  line L12 (59.4443, -3) -> (64.4443, -3) projected
  arc A15 (66.4443, -3) -> (64.4443, -3) centre (65.4443, -3) ccw projected
  line L13 (66.4443, -3) -> (66.4443, -6) projected
  arc A16 (64.4443, -6) -> (66.4443, -6) centre (65.4443, -6) ccw projected
  line L14 (64.4443, -6) -> (59.4443, -6) projected
  arc A17 (57.4443, -6) -> (59.4443, -6) centre (58.4443, -6) ccw projected
  arc A18 (89.8897, -3) -> (87.8897, -3) centre (88.8897, -3) ccw projected
  line L15 (89.8897, -3) -> (94.8897, -3) projected
  arc A19 (96.8897, -3) -> (94.8897, -3) centre (95.8897, -3) ccw projected
  line L16 (96.8897, -3) -> (96.8897, -6) projected
  arc A20 (94.8897, -6) -> (96.8897, -6) centre (95.8897, -6) ccw projected
  line L17 (94.8897, -6) -> (89.8897, -6) projected
  arc A21 (87.8897, -6) -> (89.8897, -6) centre (88.8897, -6) ccw projected
  line L18 (87.8897, -6) -> (87.8897, -3) projected
  circle A22 centre (111.885, -39) radius 1.5 projected
  arc A23 (102.2194, -50.4706) -> (121.0577, -50.8686) centre (111.885, -39) ccw projected
  line L19 (121.0577, -50.8686) -> (127.6513, -45.7727) projected
  line L20 (127.6513, -45.7727) -> (126.8081, -37.4821) projected
  arc A24 (126.8081, -37.4821) -> (124.1514, -30.3665) centre (111.885, -39) ccw projected
  line L21 (124.1514, -30.3665) -> (104.8897, -3) projected
  line L22 (104.8897, -3) -> (101.8897, -3) projected
  arc A25 (99.8897, -3) -> (101.8897, -3) centre (100.8897, -3) ccw projected
  line L23 (99.8897, -3) -> (99.8897, 0) projected
  line L24 (99.8897, 0) -> (84.8897, 0) projected
  line L25 (84.8897, 0) -> (84.8897, -3) projected
  arc A26 (82.8897, -3) -> (84.8897, -3) centre (83.8897, -3) ccw projected
  line L26 (82.8897, -3) -> (71.4443, -3) projected
  arc A27 (69.4443, -3) -> (71.4443, -3) centre (70.4443, -3) ccw projected
  line L27 (69.4443, -3) -> (69.4443, 0) projected
  line L28 (69.4443, 0) -> (54.4443, 0) projected
  line L29 (54.4443, 0) -> (54.4443, -3) projected
  arc A28 (52.4443, -3) -> (54.4443, -3) centre (53.4443, -3) ccw projected
  line L30 (52.4443, -3) -> (49.4443, -3) projected
  line L31 (49.4443, -3) -> (49.4443, -6) projected
  line L32 (49.4443, -6) -> (102.2194, -50.4706) projected
  line L33 (48.3735, -96.6751) -> (119.8722, -51.6966)
  arc A29 (102.2194, -50.4706) -> (121.0577, -50.8686) centre (111.885, -39) ccw projected
  arc A30 (102.2194, -50.4706) -> (121.0577, -50.8686) centre (111.885, -39) ccw projected
  line L34 (-20.8943, -95.75) -> (66.3014, -95.75)
  line L35 (66.3014, -95.75) -> (66.3014, -56.05)
  line L36 (66.3014, -56.05) -> (66.3014, -31.35)
  point P0 (0, 0)
  point P1 (44.6461, -83.75)
  point P2 (49.5451, -95.75)
  point P3 (66.3014, -85.397)
  point P4 (54.3014, -10.0927)
  dimension "d126" = 6
  dimension "d127" = 8
  dimension "d128" = 29
  dimension "d129" = 1
  dimension "d130" = 3
  dimension "d131" = 16
  dimension "d132" = 68
  dimension "d133" = 3
  dimension "d134" = 2
  dimension "d135" = 3
  dimension "d136" = 18
  dimension "d137" = 12
  constraints: 30 end point, 12 centre point, 4 coincident, 3 collinear, 3 horizontal, 2 vertical, 1 point on circle, 1 tangent, 13 other
  measures "d126" diameter of A3
  measures "d127" diameter of A4
  measures "d128" diameter of A5
  measures "d129" radial gap between concentric circles of A3 A6
  measures "d131" diameter of A9
  measures "d132" diameter of A11
  measures "d133" distance between parallel lines of L3 L5
  measures "d134" radial gap between concentric circles of A1 A12
  measures "d135" distance between parallel lines of L7 L8
  measures "d136" distance of A8.centre A4.centre
  measures "d137" distance between parallel lines of L8 L34
extrude "押し出し16" add sketch "スケッチ13" against normal blind 5 contours A1 L35 L36 | A1 L36 A5 L35 | L36 L35 A1 L9 L3 A11 | A1 A11 A5 L36 | L35 A5 L9 A1 | A11 L3 A1 | A1 L3 A5 A11 | L36 A12 L35 A5 | A5 A11 A12 L36 | L35 A12 L9 A5 | A5 L3 A12 A11 | A12 A11 L3 L32 A23 L33 L35 | L35 L33 L34 A7 L8 L9 A12 | A12 L3 A11 | L35 L34 L33 | A7 L34 | A7 L34 | A4
hole "穴1" at (44.6461, -90.75, 0) direction (0, 0, -1) diameter 8.05 depth 12 tip angle 118
fillet "フィレット1" radius 18 1 edges at (66.3014, -85.397, -2.5)
fillet "フィレット2" radius 1 3 edges at (54.3014, -83.75, -2.5) (49.5451, -95.75, -2.5) (54.3014, -10.0927, -2.5)
sketch "スケッチ14" plane through (0, 0, 0) normal (0, 0, 1) x (1, 0, 0)
  circle A0 centre (44.6461, -90.75) radius 4.025 projected
  line L0 (57.4443, -6) -> (57.4443, -3) projected
  arc A1 (59.4443, -3) -> (57.4443, -3) centre (58.4443, -3) ccw projected
  line L1 (59.4443, -3) -> (64.4443, -3) projected
  arc A2 (66.4443, -3) -> (64.4443, -3) centre (65.4443, -3) ccw projected
  line L2 (66.4443, -3) -> (66.4443, -6) projected
  arc A3 (64.4443, -6) -> (66.4443, -6) centre (65.4443, -6) ccw projected
  line L3 (64.4443, -6) -> (59.4443, -6) projected
  arc A4 (57.4443, -6) -> (59.4443, -6) centre (58.4443, -6) ccw projected
  arc A5 (89.8897, -3) -> (87.8897, -3) centre (88.8897, -3) ccw projected
  line L4 (89.8897, -3) -> (94.8897, -3) projected
  arc A6 (96.8897, -3) -> (94.8897, -3) centre (95.8897, -3) ccw projected
  line L5 (96.8897, -3) -> (96.8897, -6) projected
  arc A7 (94.8897, -6) -> (96.8897, -6) centre (95.8897, -6) ccw projected
  line L6 (94.8897, -6) -> (89.8897, -6) projected
  arc A8 (87.8897, -6) -> (89.8897, -6) centre (88.8897, -6) ccw projected
  line L7 (87.8897, -6) -> (87.8897, -3) projected
  circle A9 centre (111.885, -39) radius 1.5 projected
  arc A10 (119.8722, -51.6966) -> (121.0577, -50.8686) centre (111.885, -39) ccw projected
  line L8 (121.0577, -50.8686) -> (127.6513, -45.7727) projected
  line L9 (127.6513, -45.7727) -> (126.8081, -37.4821) projected
  arc A11 (126.8081, -37.4821) -> (124.1514, -30.3665) centre (111.885, -39) ccw projected
  line L10 (124.1514, -30.3665) -> (104.8897, -3) projected
  line L11 (104.8897, -3) -> (101.8897, -3) projected
  arc A12 (99.8897, -3) -> (101.8897, -3) centre (100.8897, -3) ccw projected
  line L12 (99.8897, -3) -> (99.8897, 0) projected
  line L13 (99.8897, 0) -> (84.8897, 0) projected
  line L14 (84.8897, 0) -> (84.8897, -3) projected
  arc A13 (82.8897, -3) -> (84.8897, -3) centre (83.8897, -3) ccw projected
  line L15 (82.8897, -3) -> (71.4443, -3) projected
  arc A14 (69.4443, -3) -> (71.4443, -3) centre (70.4443, -3) ccw projected
  line L16 (69.4443, -3) -> (69.4443, 0) projected
  line L17 (69.4443, 0) -> (54.4443, 0) projected
  line L18 (54.4443, 0) -> (54.4443, -3) projected
  arc A15 (52.4443, -3) -> (54.4443, -3) centre (53.4443, -3) ccw projected
  line L19 (52.4443, -3) -> (49.4443, -3) projected
  line L20 (49.4443, -3) -> (49.4443, -6) projected
  line L21 (49.4443, -6) -> (53.9457, -9.7931) projected
  arc A16 (54.3014, -10.5578) -> (53.9457, -9.7931) centre (53.3014, -10.5578) ccw projected
  line L22 (54.3014, -10.5578) -> (54.3014, -82.75) projected
  arc A17 (53.3014, -83.75) -> (54.3014, -82.75) centre (53.3014, -82.75) ccw projected
  line L23 (53.3014, -83.75) -> (44.6461, -83.75) projected
  arc A18 (44.6461, -83.75) -> (49.2762, -96) centre (44.6461, -90.75) ccw projected
  arc A19 (49.9376, -95.75) -> (49.2762, -96) centre (49.9376, -96.75) ccw projected
  line L24 (49.9376, -95.75) -> (66.3014, -95.75) projected
  line L25 (66.3014, -95.75) -> (66.3014, -95.339) projected
  arc A20 (74.7167, -80.1031) -> (66.3014, -95.339) centre (84.3014, -95.339) ccw projected
  line L26 (74.7167, -80.1031) -> (119.8722, -51.6966) projected
  point P0 (0, 0)
sketch "スケッチ15" plane through (0, 0, 0) normal (0, 0, 1) x (1, 0, 0)
  circle A0 centre (46.8822, -88.25) radius 1.5
  line L0 (45.3386, -92.477) -> (54.3014, -95.75)
  line L1 (54.3014, -95.75) -> (66.3014, -95.75)
  line L2 (66.3014, -95.75) -> (66.3014, -95.339)
  arc A1 (74.7167, -80.1031) -> (66.3014, -95.339) centre (84.3014, -95.339) ccw
  line L3 (74.7167, -80.1031) -> (119.8722, -51.6966)
  arc A2 (119.8722, -51.6966) -> (121.0577, -50.8686) centre (111.885, -39) ccw
  line L4 (121.0577, -50.8686) -> (127.6513, -45.7727)
  line L5 (127.6513, -45.7727) -> (119.127, -45.896)
  arc A3 (104.885, -31.8586) -> (119.127, -45.896) centre (111.885, -39) ccw
  line L6 (104.885, -31.8586) -> (104.885, -3)
  line L7 (104.885, -3) -> (101.8897, -3)
  arc A4 (99.8897, -3) -> (101.8897, -3) centre (100.8897, -3) ccw
  line L8 (99.8897, -3) -> (96.8897, -3)
  line L9 (96.8897, -3) -> (96.8897, -6)
  arc A5 (94.8897, -6) -> (96.8897, -6) centre (95.8897, -6) ccw
  line L10 (94.8897, -6) -> (89.8897, -6)
  arc A6 (87.8897, -6) -> (89.8897, -6) centre (88.8897, -6) ccw
  line L11 (87.8897, -6) -> (87.8897, -3)
  line L12 (87.8897, -3) -> (84.8897, -3)
  arc A7 (82.8897, -3) -> (84.8897, -3) centre (83.8897, -3) ccw
  line L13 (82.8897, -3) -> (71.4443, -3)
  arc A8 (69.4443, -3) -> (71.4443, -3) centre (70.4443, -3) ccw
  line L14 (69.4443, -3) -> (66.4443, -3)
  line L15 (66.4443, -3) -> (66.4443, -6)
  arc A9 (64.4443, -6) -> (66.4443, -6) centre (65.4443, -6) ccw
  line L16 (64.4443, -6) -> (59.4443, -6)
  arc A10 (57.4443, -6) -> (59.4443, -6) centre (58.4443, -6) ccw
  line L17 (57.4443, -6) -> (57.4443, -3)
  line L18 (57.4443, -3) -> (54.4443, -3)
  arc A11 (52.4443, -3) -> (54.4443, -3) centre (53.4443, -3) ccw
  line L19 (52.4443, -3) -> (49.4443, -3)
  line L20 (49.4443, -3) -> (49.4443, -6)
  line L21 (49.4443, -6) -> (53.9457, -9.7931)
  arc A12 (54.3014, -10.5578) -> (53.9457, -9.7931) centre (53.3014, -10.5578) ccw
  line L22 (54.3014, -10.5578) -> (54.3014, -82.75)
  arc A13 (53.3014, -83.75) -> (54.3014, -82.75) centre (53.3014, -82.75) ccw
  line L23 (53.3014, -83.75) -> (46.8822, -83.75)
  arc A14 (46.8822, -83.75) -> (45.3386, -92.477) centre (46.8822, -88.25) ccw
  circle A15 centre (44.6461, -90.75) radius 4.025 projected
  line L24 (57.4443, -6) -> (57.4443, -3) projected
  arc A16 (59.4443, -3) -> (57.4443, -3) centre (58.4443, -3) ccw projected
  line L25 (59.4443, -3) -> (64.4443, -3) projected
  arc A17 (66.4443, -3) -> (64.4443, -3) centre (65.4443, -3) ccw projected
  line L26 (66.4443, -3) -> (66.4443, -6) projected
  arc A18 (64.4443, -6) -> (66.4443, -6) centre (65.4443, -6) ccw projected
  line L27 (64.4443, -6) -> (59.4443, -6) projected
  arc A19 (57.4443, -6) -> (59.4443, -6) centre (58.4443, -6) ccw projected
  arc A20 (89.8897, -3) -> (87.8897, -3) centre (88.8897, -3) ccw projected
  line L28 (89.8897, -3) -> (94.8897, -3) projected
  arc A21 (96.8897, -3) -> (94.8897, -3) centre (95.8897, -3) ccw projected
  line L29 (96.8897, -3) -> (96.8897, -6) projected
  arc A22 (94.8897, -6) -> (96.8897, -6) centre (95.8897, -6) ccw projected
  line L30 (94.8897, -6) -> (89.8897, -6) projected
  arc A23 (87.8897, -6) -> (89.8897, -6) centre (88.8897, -6) ccw projected
  line L31 (87.8897, -6) -> (87.8897, -3) projected
  circle A24 centre (111.885, -39) radius 1.5 projected
  arc A25 (119.8722, -51.6966) -> (121.0577, -50.8686) centre (111.885, -39) ccw projected
  line L32 (121.0577, -50.8686) -> (127.6513, -45.7727) projected
  line L33 (127.6513, -45.7727) -> (126.8081, -37.4821) projected
  arc A26 (126.8081, -37.4821) -> (124.1514, -30.3665) centre (111.885, -39) ccw projected
  line L34 (124.1514, -30.3665) -> (104.8897, -3) projected
  line L35 (104.8897, -3) -> (101.8897, -3) projected
  arc A27 (99.8897, -3) -> (101.8897, -3) centre (100.8897, -3) ccw projected
  line L36 (99.8897, -3) -> (99.8897, 0) projected
  line L37 (99.8897, 0) -> (84.8897, 0) projected
  line L38 (84.8897, 0) -> (84.8897, -3) projected
  arc A28 (82.8897, -3) -> (84.8897, -3) centre (83.8897, -3) ccw projected
  line L39 (82.8897, -3) -> (71.4443, -3) projected
  arc A29 (69.4443, -3) -> (71.4443, -3) centre (70.4443, -3) ccw projected
  line L40 (69.4443, -3) -> (69.4443, 0) projected
  line L41 (69.4443, 0) -> (54.4443, 0) projected
  line L42 (54.4443, 0) -> (54.4443, -3) projected
  arc A30 (52.4443, -3) -> (54.4443, -3) centre (53.4443, -3) ccw projected
  line L43 (52.4443, -3) -> (49.4443, -3) projected
  line L44 (49.4443, -3) -> (49.4443, -6) projected
  line L45 (49.4443, -6) -> (53.9457, -9.7931) projected
  arc A31 (54.3014, -10.5578) -> (53.9457, -9.7931) centre (53.3014, -10.5578) ccw projected
  line L46 (54.3014, -10.5578) -> (54.3014, -82.75) projected
  arc A32 (53.3014, -83.75) -> (54.3014, -82.75) centre (53.3014, -82.75) ccw projected
  line L47 (53.3014, -83.75) -> (44.6461, -83.75) projected
  arc A33 (44.6461, -83.75) -> (49.2762, -96) centre (44.6461, -90.75) ccw projected
  arc A34 (49.9376, -95.75) -> (49.2762, -96) centre (49.9376, -96.75) ccw projected
  line L48 (49.9376, -95.75) -> (66.3014, -95.75) projected
  line L49 (66.3014, -95.75) -> (66.3014, -95.339) projected
  arc A35 (74.7167, -80.1031) -> (66.3014, -95.339) centre (84.3014, -95.339) ccw projected
  line L50 (74.7167, -80.1031) -> (119.8722, -51.6966) projected
  point P0 (0, 0)
  point P1 (0, 0)
  point P2 (46.0735, -86.9866)
  point P3 (48.2276, -88.9133)
  point P4 (47.7212, -93.347)
  point P5 (42.4703, -87.3638)
  constraints: 48 end point, 28 point on circle, 15 centre point, 11 horizontal, 8 vertical, 75 other
extrude "押し出し17" cut sketch "スケッチ15" against normal blind 10 contours A0 A15 | A15 L0 L48 A34 A33 L47 A14 picked at (47.4573, -87.5246)
extrude "押し出し18" add sketch "スケッチ15" against normal blind 5 contours A0 A15 L0 A14